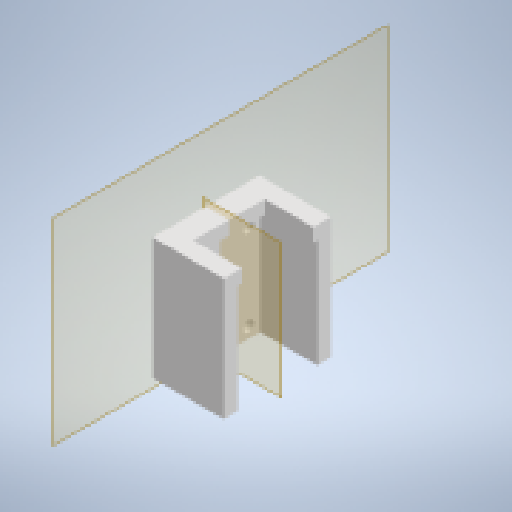
# Autodesk Inventor part: держатель магнитов на основе
Saved by Autodesk Inventor 2024.2 (Build 282272000, 272)
## iProperties
Created: 2025-12-27
Part Number: держатель магнитов на основе
Material: Типовые
Document SubType Name: Modeling
Designer: katya_notebook
Density: 1 g/cm^3
Appearance: По умолчанию
Author: katya_notebook
Autodesk Inventor part; units mm, degrees
ref_plane "YZ Plane" through (0, 0, 0) normal (1, 0, 0) x (0, 1, 0)
ref_plane "XZ Plane" through (0, 0, 0) normal (0, 1, 0) x (-1, 0, 0)
sketch "Эскиз1" plane through (0, 0, 0) normal (1, 0, 0) x (0, 1, 0)
  line L0 (-15, -10.95) -> (15, -10.95)
  line L1 (15, -10.95) -> (15, 10.95)
  line L2 (15, 10.95) -> (-15, 10.95)
  line L3 (-15, 10.95) -> (-15, -10.95)
  line L4 (-15, -10.95) -> (15, 10.95) construction
  line L5 (15, -10.95) -> (-15, 10.95) construction
  circle A0 centre (7, 0) radius 5
  circle A1 centre (-7, 0) radius 5
  point P0 (0, 0)
  dimension "d0" = 30
  dimension "d1" = 21.9
  dimension "d2" = 10
  dimension "d3" = 10
  dimension "d4" = 8
  dimension "d5" = 14
  dimension "d6" = 8
  dimension "d7" = 0
  constraints: 12 end point, 2 centre point, 2 midpoint, 2 parallel, 1 horizontal, 1 perpendicular
  measures "d0" distance of L1.end L2.end
  measures "d1" distance of L0.end L1.end
  measures "d2" diameter of A0
  measures "d3" diameter of A1
  measures "d4" distance from line of A0.centre L1
  measures "d5" distance of A1.centre A0.centre
  measures "d6" distance from line of L3 A1.centre
  measures "d7" vertical distance of point (0, 0) A0.centre
extrude "Выдавливание1" add sketch "Эскиз1" along normal blind 2
sketch "Эскиз2" plane through (2, 0, 0) normal (1, 0, 0) x (0, 0, -1)
  line L0 (10.95, 15) -> (-10.95, 15) projected
  line L1 (10.95, -15) -> (-10.95, -15)
  line L2 (-10.95, -15) -> (-10.95, 15)
  line L3 (-10.95, 15) -> (10.95, 15)
  line L4 (10.95, 15) -> (10.95, -15)
  line L5 (10.95, -15) -> (-10.95, 15) construction
  line L6 (-10.95, -15) -> (10.95, 15) construction
  point P0 (0, 0)
  constraints: 12 end point, 2 midpoint, 2 parallel, 1 horizontal, 1 perpendicular
extrude "Выдавливание2" add sketch "Эскиз2" along normal blind 2
sketch "Эскиз3" plane through (0, 0, 0) normal (-1, 0, 0) x (0, 0, 1)
  circle A0 centre (-7.95, 12) radius 1.5
  line L0 (-10.95, 15) -> (10.95, 15) projected
  line L1 (-10.95, -15) -> (-10.95, 15) projected
  circle A1 centre (-7.95, -12) radius 1.5
  line L2 (10.95, -15) -> (-10.95, -15) projected
  circle A2 centre (7.95, 12) radius 1.5
  line L3 (10.95, 15) -> (10.95, -15) projected
  circle A3 centre (7.95, -12) radius 1.5
  point P0 (0, 0)
  dimension "d12" = 3
  dimension "d13" = 3
  dimension "d14" = 3
  dimension "d15" = 3
  dimension "d16" = 3
  dimension "d17" = 3
  dimension "d18" = 3
  dimension "d19" = 3
  dimension "d20" = 3
  constraints: 4 centre point
  measures "d12" diameter of A0
  measures "d13" distance from line of L0 A0.centre
  measures "d14" distance from line of L1 A0.centre
  measures "d15" diameter of A1
  measures "d16" distance from line of L1 A1.centre
  measures "d17" distance from line of L2 A1.centre
  measures "d18" diameter of A2
  measures "d19" distance from line of L3 A2.centre
  measures "d20" diameter of A3
extrude "Выдавливание3" cut sketch "Эскиз3" against normal up to surface (4 mm away) contours A0 | A1 | A2 | A3
ref_plane "РабПлоскость1" through (0, 10, -4) normal (1, 0, 0) x (0, 0, -1)
sketch "Эскиз4" plane through (0, 10, -4) normal (1, 0, 0) x (0, 0, -1)
  line L0 (6.95, 5) -> (-14.95, 5) projected
  line L1 (-14.95, 5) -> (6.95, 5)
  line L2 (6.95, 5) -> (6.95, 9)
  line L3 (6.95, 9) -> (-14.95, 9)
  line L4 (-14.95, 9) -> (-14.95, 5)
  point P0 (-4, -10)
  dimension "d23" = 4
  constraints: 8 end point, 2 parallel, 1 horizontal, 1 perpendicular
  measures "d23" distance of L3.end L0.end
extrude "Выдавливание4" add sketch "Эскиз4" along normal blind 6.5
sketch "Эскиз5" plane through (4, -15, -10.95) normal (0, 0, -1) x (-1, 0, 0)
  line L0 (4, 34) -> (4, 0) projected
  line L1 (4, 34) -> (-16, 34)
  line L2 (-16, 34) -> (-16, 0)
  line L3 (-16, 0) -> (4, 0)
  line L4 (4, 0) -> (4, 34)
  point P0 (4, 15)
  dimension "d26" = 20
  constraints: 8 end point, 2 parallel, 1 horizontal, 1 perpendicular
  measures "d26" distance of L0.start L1.end
extrude "Выдавливание5" add sketch "Эскиз5" along normal blind 4
sketch "Эскиз6" plane through (0, -15, 10.95) normal (0, 0, 1) x (1, 0, 0)
  line L0 (0, 0) -> (0, 34) projected
  line L1 (20, 34) -> (20, 0) projected
  line L2 (0, 0) -> (20, 0)
  line L3 (20, 0) -> (20, 34)
  line L4 (20, 34) -> (0, 34)
  line L5 (0, 34) -> (0, 0)
  point P0 (0, 15)
  point P1 (20, 0)
  point P2 (0, 34)
  constraints: 8 end point, 2 parallel, 1 horizontal, 1 perpendicular
extrude "Выдавливание6" add sketch "Эскиз6" along normal blind 4
sketch "Эскиз7" plane through (0, -15, 10.95) normal (0, 0, -1) x (-1, 0, 0)
  line L0 (-20, 0) -> (-20, 34) projected
  line L1 (-20, 0) -> (-4, 0)
  line L2 (-4, 0) -> (-4, 30)
  line L3 (-4, 30) -> (-20, 30)
  line L4 (-20, 30) -> (-20, 0)
  point P0 (0, 15)
  constraints: 8 end point, 2 parallel, 1 horizontal, 1 perpendicular
extrude "Выдавливание7" cut sketch "Эскиз7" along normal mid plane 0.2
sketch "Эскиз8" plane through (4, -15, -10.95) normal (0, 0, 1) x (1, 0, 0)
  line L0 (16, 34) -> (16, 0) projected
  line L1 (0, 0) -> (0, 30) projected
  line L2 (16, 0) -> (0, 0)
  line L3 (0, 0) -> (0, 30)
  line L4 (0, 30) -> (16, 30)
  line L5 (16, 30) -> (16, 0)
  point P0 (-4, 15)
  constraints: 8 end point, 2 parallel, 1 horizontal, 1 perpendicular
extrude "Выдавливание8" cut sketch "Эскиз8" against normal blind 0.2
sketch "Эскиз9" plane through (0, -15, 10.95) normal (0, 0, -1) x (-1, 0, 0)
  line L0 (-20, 30) -> (-6.5, 30) projected
  line L1 (-6.5, 34) -> (-20, 34)
  line L2 (-20, 34) -> (-20, 30)
  line L3 (-20, 30) -> (-6.5, 30)
  line L4 (-6.5, 30) -> (-6.5, 34)
  point P0 (0, 15)
  constraints: 8 end point, 2 parallel, 1 horizontal, 1 perpendicular
extrude "Выдавливание9" add sketch "Эскиз9" along normal blind 1
sketch "Эскиз10" plane through (4, -15, -10.95) normal (0, 0, 1) x (1, 0, 0)
  line L0 (2.5, 30) -> (2.5, 34) projected
  line L1 (2.5, 30) -> (16, 30) projected
  line L2 (2.5, 34) -> (16, 34)
  line L3 (16, 34) -> (16, 30)
  line L4 (16, 30) -> (2.5, 30)
  line L5 (2.5, 30) -> (2.5, 34)
  point P0 (-4, 15)
  constraints: 8 end point, 2 parallel, 1 horizontal, 1 perpendicular
extrude "Выдавливание10" add sketch "Эскиз10" along normal blind 1
sketch "Эскиз11" plane through (4, 15, 11.05) normal (0, -1, 0) x (1, 0, 0)
  line L0 (0, -22.2) -> (0, 0) projected
  line L1 (0, -22.2) -> (16, -22.2) projected
  line L2 (16, -22.2) -> (16, -21) projected
  line L3 (2.5, -21) -> (16, -21) projected
  line L4 (2.5, -1.1) -> (2.5, -21) projected
  line L5 (16, -1.1) -> (2.5, -1.1) projected
  line L6 (16, 0) -> (16, -1.1) projected
  line L7 (16, 0) -> (0, 0) projected
  point P0 (-4, -11.05)
extrude "Выдавливание11" cut sketch "Эскиз11" against normal blind 0.2
